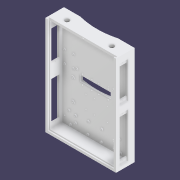
# Autodesk Inventor part: BP001b
Saved by Autodesk Inventor 2017 SP1 (Build 210196100, 196)
## iProperties
Created: 2017-12-18
Part Number: BP001b
Material: ABS Plastic
Document SubType Name: Modeling
Designer: Zach
Density: 1.06 g/cm^3
Appearance: CR White
Author: Zach
Autodesk Inventor part; units mm, degrees
ref_plane "YZ Plane" through (0, 0, 0) normal (1, 0, 0) x (0, 1, 0)
ref_plane "XZ Plane" through (0, 0, 0) normal (0, 1, 0) x (-1, 0, 0)
ref_plane "XY Plane" through (0, 0, 0) normal (0, 0, 1) x (1, 0, 0)
sketch "Sketch1" plane through (0, 0, 0) normal (0, 0, 1) x (1, 0, 0)
  line L0 (0, 0) -> (130, 0)
  line L1 (130, 0) -> (130, 25)
  line L2 (130, 25) -> (0, 25)
  line L3 (0, 25) -> (0, 0)
  line L4 (10.3559, 32.5) -> (50.3559, 32.5) construction
  line L5 (50.3559, 32.5) -> (50.3559, -7.5) construction
  line L6 (50.3559, -7.5) -> (10.3559, -7.5) construction
  line L7 (10.3559, -7.5) -> (10.3559, 32.5) construction
  line L8 (79.6441, 32.5) -> (119.6441, 32.5) construction
  line L9 (119.6441, 32.5) -> (119.6441, -7.5) construction
  line L10 (119.6441, -7.5) -> (79.6441, -7.5) construction
  line L11 (79.6441, -7.5) -> (79.6441, 32.5) construction
  line L12 (50.3559, 12.5) -> (79.6441, 12.5) construction
  circle A0 centre (10.3559, 32.5) radius 2.5
  circle A1 centre (50.3559, 32.5) radius 2.5
  circle A2 centre (50.3559, -7.5) radius 2.5
  circle A3 centre (10.3559, -7.5) radius 2.5
  circle A4 centre (79.6441, -7.5) radius 2.5
  circle A5 centre (119.6441, -7.5) radius 2.5
  circle A6 centre (119.6441, 32.5) radius 2.5
  circle A7 centre (79.6441, 32.5) radius 2.5
  line L13 (-85, -197.5) -> (215, -197.5)
  line L14 (215, -197.5) -> (215, 222.5)
  line L15 (215, 222.5) -> (-85, 222.5)
  line L16 (-85, 222.5) -> (-85, -197.5)
  point P0 (130, 12.5)
  point P1 (65, 12.5)
  point P2 (65, 25)
  point P3 (215, 12.5)
  point P4 (65, 222.5)
  dimension "d0" = 130
  dimension "d1" = 25
  dimension "d2" = 40
  dimension "d3" = 40
  dimension "d4" = 40
  dimension "d5" = 40
  dimension "d6" = 29.2883
  dimension "d7" = 5
  dimension "d8" = 5
  dimension "d9" = 5
  dimension "d10" = 5
  dimension "d11" = 5
  dimension "d12" = 5
  dimension "d13" = 5
  dimension "d14" = 5
  dimension "d15" = 300
  dimension "d16" = 420
  constraints: 34 end point, 8 centre point, 8 coincident, 8 parallel, 7 midpoint, 4 horizontal, 4 perpendicular, 2 horizontal alignment, 2 vertical alignment, 1 point on line
  measures "d0" distance of L2.end L1.end
  measures "d1" distance of L1.end L0.end
  measures "d2" distance of L5.end L6.end
  measures "d3" distance of L4.end L5.end
  measures "d4" distance of L9.end L10.end
  measures "d5" distance of L8.end L9.end
  measures "d6" distance between parallel lines of L11 L5
  measures "d7" diameter of A0
  measures "d8" diameter of A1
  measures "d9" diameter of A2
  measures "d10" diameter of A3
  measures "d11" diameter of A4
  measures "d12" diameter of A5
  measures "d13" diameter of A6
  measures "d14" diameter of A7
  measures "d15" distance of L15.end L14.end
  measures "d16" distance of L14.end L13.end
extrude "Extrusion1" add sketch "Sketch1" along normal blind 17
sketch "Sketch2" plane through (0, 0, 17) normal (0, 0, 1) x (1, 0, 0)
  line L0 (-85, 222.5) -> (-85, -197.5) projected
  line L1 (215, 222.5) -> (-85, 222.5) projected
  line L2 (215, -197.5) -> (215, 222.5) projected
  line L3 (-85, -197.5) -> (215, -197.5) projected
  line L4 (-75, -187.5) -> (-75, 212.5)
  line L5 (-75, 212.5) -> (205, 212.5)
  line L6 (205, 212.5) -> (205, -187.5)
  line L7 (205, -187.5) -> (-75, -187.5)
  point P0 (0, 0)
  dimension "d19" = 10
  constraints: 8 end point, 3 other
  measures "d19" distance between parallel lines of L0 L4
extrude "Extrusion2" add sketch "Sketch2" along normal blind 52
sketch "Sketch3" plane through (-85, 222.5, 0) normal (0, 1, 0) x (1, 0, 0)
  line L0 (0, 0) -> (300, 0) construction
  line L1 (70, 0) -> (230, 0)
  arc A0 (70, 0) -> (230, 0) centre (150, 304.672) ccw
  point P0 (85, 0)
  point P1 (150, 0)
  dimension "d23" = 160
  dimension "d24" = 315
  constraints: 2 end point, 2 midpoint, 2 point on circle, 2 point on line, 1 centre point
  measures "d23" distance of L1.start L1.end
  measures "d24" radius of A0
extrude "Extrusion3" cut sketch "Sketch3" against normal through all
sketch "Sketch5" plane through (0, 0, 17) normal (0, 0, 1) x (1, 0, 0)
  line L0 (-12.46, 197.48) -> (142.46, 197.48) construction
  line L1 (142.46, 197.48) -> (142.46, 40) construction
  line L2 (142.46, 40) -> (-12.46, 40) construction
  line L3 (-12.46, 40) -> (-12.46, 197.48) construction
  line L4 (0, 25) -> (130, 25) construction
  line L5 (-75, 212.5) -> (205, 212.5) construction
  circle A0 centre (142.46, 197.48) radius 1.5
  circle A1 centre (142.46, 40) radius 1.5
  circle A2 centre (-12.46, 40) radius 1.5
  circle A3 centre (-12.46, 197.48) radius 1.5
  circle A4 centre (25.3559, -90.75) radius 1.5
  circle A5 centre (25.3559, -34.25) radius 1.5
  line L6 (130, 0) -> (0, 0) construction
  line L7 (65, 0) -> (65, -187.5) construction
  line L8 (-75, -187.5) -> (205, -187.5) projected
  line L9 (-75, -187.5) -> (-75, 212.5) projected
  line L10 (205, 212.5) -> (205, -187.5) projected
  line L11 (160, -90) -> (160, 0) construction
  circle A6 centre (160, 0) radius 1.5
  circle A7 centre (160, -90) radius 1.5
  line L12 (-30, 0) -> (-30, -90) construction
  circle A8 centre (-30, 0) radius 1.5
  circle A9 centre (-30, -90) radius 1.5
  circle A10 centre (119.62, 40) radius 1.5
  line L13 (60.3559, -92.5) -> (116.8559, -92.5) construction
  circle A11 centre (116.8559, -92.5) radius 1.5
  circle A12 centre (60.3559, -92.5) radius 1.5
  line L14 (60.3559, -32.5) -> (116.8559, -32.5) construction
  circle A13 centre (116.8559, -32.5) radius 1.5
  circle A14 centre (60.3559, -32.5) radius 1.5
  circle A15 centre (50.3559, -7.5) radius 2.5 construction
  line L15 (25.3559, -34.25) -> (25.3559, -90.75) construction
  line L16 (88.6059, -92.5) -> (88.6059, -32.5) construction
  point P0 (65, 40)
  point P1 (65, -93.75)
  point P2 (65, -80)
  point P3 (88.6059, -62.5)
  point P4 (25.3559, -62.5)
  dimension "d27" = 154.92
  dimension "d28" = 157.48
  dimension "d29" = 3
  dimension "d30" = 3
  dimension "d31" = 3
  dimension "d32" = 3
  dimension "d34" = 3
  dimension "d35" = 3
  dimension "d112" = 45
  dimension "d115" = 3
  dimension "d116" = 3
  dimension "d117" = 45
  dimension "d118" = 3
  dimension "d119" = 3
  dimension "d129" = 90
  dimension "d131" = 0
  dimension "d239" = 3
  dimension "d240" = 22.84
  dimension "d241" = 15
  dimension "d260" = 56.5
  dimension "d261" = 3
  dimension "d262" = 3
  dimension "d263" = 56.5
  dimension "d264" = 3
  dimension "d265" = 3
  dimension "d266" = 10
  dimension "d267" = 25
  dimension "d268" = 60
  dimension "d269" = 56.5
  dimension "d270" = 35
  constraints: 22 end point, 15 centre point, 12 coincident, 11 midpoint, 4 vertical alignment, 3 horizontal, 3 horizontal alignment, 3 vertical, 2 parallel, 1 perpendicular, 1 point on line
  measures "d27" distance of L1.end L2.end
  measures "d28" distance of L0.end L1.end
  measures "d29" diameter of A0
  measures "d30" diameter of A1
  measures "d31" diameter of A2
  measures "d32" diameter of A3
  measures "d34" diameter of A4
  measures "d35" diameter of A5
  measures "d112" distance between parallel lines of L10 L11
  measures "d115" diameter of A6
  measures "d116" diameter of A7
  measures "d117" distance between parallel lines of L9 L12
  measures "d118" diameter of A8
  measures "d119" diameter of A9
  measures "d129" distance of A6.centre L11.start
  measures "d131" distance from line of L11.end L6
  measures "d239" diameter of A10
  measures "d240" distance from line of L1 A10.centre
  measures "d241" distance between parallel lines of L4 L2
  measures "d260" distance of L13.start L13.end
  measures "d261" diameter of A11
  measures "d262" diameter of A12
  measures "d263" distance of L14.start L14.end
  measures "d264" diameter of A13
  measures "d265" diameter of A14
  measures "d266" horizontal distance of A15.centre L14.start
  measures "d267" vertical distance of A15.centre L14.end
  measures "d268" distance between parallel lines of L13 L14
  measures "d269" distance of L15.end L15.start
  measures "d270" distance from line of L14.start L15
extrude "Extrusion4" cut sketch "Sketch5" against normal through all
sketch "Sketch6" plane through (0, 0, 17) normal (0, 0, 1) x (1, 0, 0)
  circle A0 centre (-12.46, 197.48) radius 1.5 projected
  line L0 (205, 212.5) -> (-75, 212.5) projected
  line L1 (-75, 212.5) -> (-75, -187.5) projected
  line L2 (-75, -187.5) -> (205, -187.5) projected
  line L3 (205, -187.5) -> (205, 212.5) projected
  line L4 (0, 0) -> (0, 25) projected
  line L5 (0, 25) -> (130, 25) projected
  line L6 (130, 25) -> (130, 0) projected
  line L7 (130, 0) -> (0, 0) projected
  circle A1 centre (79.6441, 32.5) radius 2.5 projected
  circle A2 centre (119.6441, 32.5) radius 2.5 projected
  circle A3 centre (119.6441, -7.5) radius 2.5 projected
  circle A4 centre (79.6441, -7.5) radius 2.5 projected
  circle A5 centre (10.3559, -7.5) radius 2.5 projected
  circle A6 centre (50.3559, -7.5) radius 2.5 projected
  circle A7 centre (50.3559, 32.5) radius 2.5 projected
  circle A8 centre (10.3559, 32.5) radius 2.5 projected
  circle A9 centre (-12.46, 197.48) radius 5
  circle A10 centre (142.46, 197.48) radius 1.5 projected
  circle A11 centre (142.46, 197.48) radius 5
  circle A12 centre (142.46, 40) radius 5
  circle A13 centre (-12.46, 40) radius 1.5 projected
  circle A14 centre (-12.46, 40) radius 5
  circle A15 centre (142.46, 40) radius 1.5 projected
  circle A16 centre (-30, 0) radius 1.5 projected
  circle A17 centre (-30, -90) radius 1.5 projected
  circle A18 centre (160, 0) radius 1.5 projected
  circle A19 centre (160, -90) radius 1.5 projected
  circle A20 centre (-30, 0) radius 1.5 projected
  circle A21 centre (-30, 0) radius 7.5
  circle A22 centre (-30, -90) radius 7.5
  circle A23 centre (160, 0) radius 7.5
  circle A24 centre (160, -90) radius 7.5
  circle A25 centre (119.62, 40) radius 1.5 projected
  circle A26 centre (119.62, 40) radius 5
  dimension "d58" = 10
  dimension "d59" = 10
  dimension "d60" = 10
  dimension "d61" = 10
  dimension "d120" = 15
  dimension "d121" = 15
  dimension "d122" = 15
  dimension "d123" = 15
  dimension "d242" = 10
  constraints: 9 centre point, 9 coincident
  measures "d58" diameter of A9
  measures "d59" diameter of A11
  measures "d60" diameter of A12
  measures "d61" diameter of A14
  measures "d120" diameter of A21
  measures "d121" diameter of A22
  measures "d122" diameter of A23
  measures "d123" diameter of A24
  measures "d242" diameter of A26
extrude "Extrusion5" add sketch "Sketch6" along normal blind 3 contours A9 | A11 | A12 | A14 | A21 | A22 | A23 | A24
sketch "Sketch7" plane through (-75, -187.5, 17) normal (1, 0, 0) x (0, 0, -1)
  line L0 (-3, 389.98) -> (-3, 379.98) projected
  line L1 (-3, 232.5) -> (-3, 222.5) projected
  line L2 (-3, 379.98) -> (-3, 232.5)
  line L3 (-12, 368.24) -> (-47, 368.24)
  line L4 (-47, 368.24) -> (-47, 244.24)
  line L5 (-47, 244.24) -> (-12, 244.24)
  line L6 (-12, 244.24) -> (-12, 368.24)
  line L7 (0, 180) -> (0, 195) projected
  line L8 (0, 180) -> (0, 195) projected
  line L9 (0, 222.5) -> (0, 232.5) projected
  line L10 (0, 379.98) -> (0, 389.98) projected
  line L11 (0, 379.98) -> (0, 389.98) projected
  line L12 (0, 222.5) -> (0, 232.5) projected
  line L13 (0, 90) -> (0, 105) projected
  line L14 (0, 90) -> (0, 105) projected
  line L15 (0, 400) -> (0, 0) projected
  line L16 (0, 0) -> (0, 400) projected
  line L17 (0, 187.5) -> (0, 212.5) projected
  line L18 (0, 212.5) -> (0, 187.5) projected
  line L19 (0, 217.5) -> (0, 222.5) projected
  line L20 (0, 217.5) -> (0, 222.5) projected
  line L21 (0, 177.5) -> (0, 182.5) projected
  line L22 (0, 177.5) -> (0, 182.5) projected
  line L23 (0, 177.5) -> (0, 182.5) projected
  line L24 (0, 177.5) -> (0, 182.5) projected
  line L25 (0, 217.5) -> (0, 222.5) projected
  line L26 (0, 217.5) -> (0, 222.5) projected
  line L27 (17, 410) -> (17, -10) projected
  point P0 (17, 187.5)
  point P1 (-47, 306.24)
  point P2 (-3, 306.24)
  point P3 (0, 106)
  point P4 (0, 109)
  point P5 (0, 106)
  point P6 (0, 109)
  point P7 (0, 146)
  point P8 (0, 149)
  point P9 (0, 146)
  point P10 (0, 149)
  point P11 (0, 98)
  point P12 (0, 101)
  point P13 (0, 98)
  point P14 (0, 101)
  dimension "d124" = 35
  dimension "d125" = 124
  dimension "d259" = 29
  constraints: 10 end point, 2 midpoint, 2 parallel, 1 horizontal, 1 horizontal alignment, 1 perpendicular, 1 vertical
  measures "d124" distance of L5.end L4.end
  measures "d125" distance of L4.end L3.end
  measures "d259" distance between parallel lines of L27 L6
extrude "Extrusion6" cut sketch "Sketch7" against normal through all
sketch "Sketch8" plane through (-85, -197.5, 0) normal (-1, 0, 0) x (0, 0, 1)
  line L0 (64, 378.24) -> (29, 378.24)
  line L1 (29, 378.24) -> (29, 393.24)
  line L2 (29, 393.24) -> (64, 393.24)
  line L3 (64, 393.24) -> (64, 378.24)
  line L4 (64, 254.24) -> (29, 254.24)
  line L5 (29, 254.24) -> (29, 239.24)
  line L6 (29, 239.24) -> (64, 239.24)
  line L7 (64, 239.24) -> (64, 254.24)
  line L8 (29, 378.24) -> (64, 378.24) projected
  line L9 (64, 254.24) -> (29, 254.24) projected
  line L10 (29, 254.24) -> (29, 378.24) projected
  point P0 (0, 187.5)
  point P1 (29, 385.74)
  point P2 (29, 246.74)
  dimension "d73" = 15
  dimension "d74" = 15
  constraints: 16 end point, 4 parallel, 2 horizontal, 2 midpoint, 2 perpendicular, 1 vertical alignment
  measures "d73" distance of L0.end L1.end
  measures "d74" distance of L4.end L5.end
extrude "Extrusion7" cut sketch "Sketch8" against normal blind 5
sketch "Sketch9" plane through (-80, -197.5, 0) normal (-1, 0, 0) x (0, 0, 1)
  circle A0 centre (46.5, 246.74) radius 1.5
  line L0 (29, 239.24) -> (29, 254.24) projected
  line L1 (64, 239.24) -> (29, 239.24) projected
  line L2 (64, 254.24) -> (64, 239.24) projected
  line L3 (29, 393.24) -> (64, 393.24) projected
  line L4 (64, 393.24) -> (64, 378.24) projected
  line L5 (29, 393.24) -> (64, 393.24) projected
  line L6 (29, 378.24) -> (29, 393.24) projected
  circle A1 centre (46.5, 385.74) radius 1.5
  line L7 (64, 378.24) -> (29, 378.24) projected
  line L8 (29, 254.24) -> (64, 254.24) projected
  line L9 (64, 378.24) -> (29, 378.24) projected
  point P0 (0, 197.5)
  point P1 (29, 246.74)
  point P2 (29, 385.74)
  point P3 (46.5, 378.24)
  point P4 (46.5, 254.24)
  point P5 (46.5, 378.24)
  dimension "d77" = 3
  dimension "d78" = 3
  constraints: 4 midpoint, 3 vertical alignment, 2 centre point, 2 horizontal alignment
  measures "d77" diameter of A0
  measures "d78" diameter of A1
extrude "Extrusion8" cut sketch "Sketch9" against normal through all contours A0 | A1
sketch "Sketch10" plane through (215, -197.5, 0) normal (1, 0, 0) x (0, 0, -1)
  circle A0 centre (-46.5, 246.74) radius 1.5 projected
  line L0 (-29, 239.24) -> (-29, 254.24) projected
  line L1 (-64, 239.24) -> (-29, 239.24) projected
  line L2 (-64, 254.24) -> (-64, 239.24) projected
  line L3 (-29, 254.24) -> (-64, 254.24) projected
  circle A1 centre (-46.5, 385.74) radius 1.5 projected
  line L4 (-29, 378.24) -> (-29, 393.24) projected
  line L5 (-64, 378.24) -> (-29, 378.24) projected
  line L6 (-64, 393.24) -> (-64, 378.24) projected
  line L7 (-29, 393.24) -> (-64, 393.24) projected
  point P0 (0, 187.5)
extrude "Extrusion9" cut sketch "Sketch10" against normal blind 5
sketch "Sketch13" plane through (205, -187.5, 17) normal (-1, 0, 0) x (0, 0, 1)
  line L0 (47, 368.24) -> (12, 368.24) projected
  line L1 (47, 383.24) -> (47, 229.24) projected
  line L2 (12, 229.24) -> (12, 383.24) projected
  line L3 (12, 244.24) -> (47, 244.24) projected
  line L4 (12, 368.24) -> (47, 368.24)
  line L5 (47, 368.24) -> (47, 244.24)
  line L6 (47, 244.24) -> (12, 244.24)
  line L7 (12, 244.24) -> (12, 368.24)
  constraints: 8 end point, 2 parallel, 1 horizontal, 1 perpendicular
extrude "Extrusion12" cut sketch "Sketch13" against normal through all
sketch "Sketch14" plane through (-85, 222.5, 69) normal (0, 1, 0) x (1, 0, 0)
  line L0 (290, 52) -> (10, 52) projected
  circle A0 centre (55, 27) radius 10
  line L1 (150, 52) -> (150, -9.8542)
  circle A1 centre (245, 27) radius 10
  point P0 (85, 69)
  dimension "d99" = 20
  dimension "d100" = 25
  dimension "d103" = 95
  dimension "d279" = 20
  dimension "d280" = 95
  constraints: 2 centre point, 2 end point, 1 horizontal alignment, 1 midpoint, 1 vertical
  measures "d99" diameter of A0
  measures "d100" distance from line of L0 A0.centre
  measures "d103" distance from line of L1 A0.centre
  measures "d279" diameter of A1
  measures "d280" distance from line of A1.centre L1
extrude "Extrusion13" cut sketch "Sketch14" against normal blind 25
sketch "Sketch18" plane through (0, 0, 17) normal (0, 0, 1) x (1, 0, 0)
  circle A0 centre (174, -176.5) radius 1.5
  circle A1 centre (146, -171) radius 1.5
  circle A2 centre (146, -143.6) radius 1.5
  circle A3 centre (167.5, -128.1) radius 1.5
  circle A4 centre (93.5, -128.1) radius 1.5
  circle A5 centre (92, -176.5) radius 1.5
  line L0 (205, -187.5) -> (-75, -187.5) projected
  line L1 (205, 212.5) -> (205, -187.5) projected
  circle A6 centre (-17.5, -133.6) radius 1.5
  circle A7 centre (-17.5, -161) radius 1.5
  circle A8 centre (35, -176.5) radius 1.5
  circle A9 centre (36.5, -128.1) radius 1.5
  circle A10 centre (-39, -176.5) radius 1.5
  circle A11 centre (-45.5, -128.1) radius 1.5
  line L2 (-75, -187.5) -> (-75, 212.5) projected
  line L3 (130, 0) -> (0, 0) projected
  line L4 (65, 0) -> (65, -187.5) construction
  line L5 (36.5, -128.1) -> (65, -128.1) construction
  line L6 (93.5, -128.1) -> (65, -128.1) construction
  dimension "d169" = 82
  dimension "d170" = 48.4
  dimension "d171" = 1.5
  dimension "d172" = 15.5
  dimension "d173" = 27.4
  dimension "d174" = 48.4
  dimension "d175" = 6.5
  dimension "d176" = 74
  dimension "d177" = 5.5
  dimension "d178" = 28
  dimension "d179" = 3
  dimension "d180" = 3
  dimension "d181" = 3
  dimension "d182" = 3
  dimension "d183" = 3
  dimension "d184" = 3
  dimension "d185" = 11
  dimension "d186" = 31
  dimension "d189" = 82
  dimension "d190" = 48.4
  dimension "d191" = 1.5
  dimension "d192" = 15.5
  dimension "d193" = 27.4
  dimension "d194" = 48.4
  dimension "d195" = 6.5
  dimension "d196" = 74
  dimension "d197" = 5.5
  dimension "d198" = 28
  dimension "d199" = 3
  dimension "d200" = 3
  dimension "d201" = 3
  dimension "d202" = 3
  dimension "d203" = 3
  dimension "d204" = 3
  constraints: 12 centre point, 6 end point, 2 coincident, 2 midpoint, 1 collinear, 1 horizontal alignment, 1 perpendicular, 1 point on line
  measures "d169" distance of A5.centre A0.centre
  measures "d170" vertical distance of L6.start A5.centre
  measures "d171" horizontal distance of A5.centre L6.start
  measures "d172" vertical distance of A2.centre L6.start
  measures "d173" distance of A1.centre A2.centre
  measures "d174" vertical distance of A3.centre A0.centre
  measures "d175" horizontal distance of A0.centre A3.centre
  measures "d176" distance of L6.start A3.centre
  measures "d177" vertical distance of A1.centre A0.centre
  measures "d178" horizontal distance of A0.centre A1.centre
  measures "d179" diameter of A0
  measures "d180" diameter of A3
  measures "d181" diameter of A2
  measures "d182" diameter of A1
  measures "d183" diameter of A5
  measures "d184" diameter of A4
  measures "d185" distance from line of L0 A0.centre
  measures "d186" distance from line of A0.centre L1
  measures "d189" distance of A9.centre A11.centre
  measures "d190" vertical distance of A8.centre A9.centre
  measures "d191" horizontal distance of A9.centre A8.centre
  measures "d192" vertical distance of A7.centre A8.centre
  measures "d193" distance of A6.centre A7.centre
  measures "d194" vertical distance of A10.centre A11.centre
  measures "d195" horizontal distance of A11.centre A10.centre
  measures "d196" distance of A8.centre A10.centre
  measures "d197" vertical distance of A6.centre A11.centre
  measures "d198" horizontal distance of A11.centre A6.centre
  measures "d199" diameter of A11
  measures "d200" diameter of A10
  measures "d201" diameter of A7
  measures "d202" diameter of A6
  measures "d203" diameter of A9
  measures "d204" diameter of A8
extrude "Extrusion16" cut sketch "Sketch18" against normal through all
sketch "Sketch20" plane through (0, 0, 69) normal (0, 0, 1) x (1, 0, 0)
  line L0 (-85, 222.5) -> (-85, -197.5) projected
  line L1 (-85, -197.5) -> (215, -197.5) projected
  line L2 (215, -197.5) -> (215, 222.5) projected
  line L3 (-80, 222.5) -> (-80, -192.5)
  line L4 (-80, -192.5) -> (210, -192.5)
  line L5 (210, -192.5) -> (210, 222.5)
  line L6 (215, 222.5) -> (-85, 222.5) projected
  line L7 (-85, 222.5) -> (-80, 222.5)
  line L8 (215, 222.5) -> (210, 222.5)
  point P0 (0, 0)
  dimension "d214" = 5
  constraints: 10 end point, 2 collinear, 2 other
  measures "d214" distance between parallel lines of L0 L3
extrude "Extrusion18" add sketch "Sketch20" along normal blind 5 contours L6 L3 L4 L5 L2 L1 L0
sketch "Sketch21" plane through (0, 0, 74) normal (0, 0, 1) x (1, 0, 0)
  line L0 (-80, -192.5) -> (-80, 222.5) projected
  line L1 (215, -197.5) -> (215, 222.5) projected
  line L2 (210, 222.5) -> (210, -192.5) projected
  line L3 (-85, 222.5) -> (-85, -197.5) projected
  line L4 (-85, 222.5) -> (-85, -197.5) projected
  line L5 (-85, -197.5) -> (215, -197.5) projected
  line L6 (215, -197.5) -> (215, 222.5) projected
  line L7 (215, 222.5) -> (210, 222.5) projected
  line L8 (210, 222.5) -> (210, -192.5) projected
  line L9 (210, -192.5) -> (-80, -192.5) projected
  line L10 (-80, -192.5) -> (-80, 222.5) projected
  line L11 (-80, 222.5) -> (-85, 222.5) projected
  line L12 (-75, -187.5) -> (-75, 212.5) projected
  line L13 (205, 212.5) -> (205, -187.5) projected
  line L14 (205, -187.5) -> (-75, -187.5) projected
  line L15 (-75, -187.5) -> (-75, -192.5)
  line L16 (205, -187.5) -> (205, -192.5)
  line L17 (-75, 212.5) -> (-75, 222.5)
  line L18 (210, 222.5) -> (-80, 222.5) projected
  line L19 (-75, 222.5) -> (-80, 222.5)
  line L20 (205, 212.5) -> (205, 222.5)
  line L21 (215, 222.5) -> (210, 222.5) projected
  line L22 (205, 222.5) -> (210, 222.5)
  line L23 (-80, -192.5) -> (210, -192.5) projected
  line L24 (205, -192.5) -> (210, -192.5)
  line L25 (-75, -192.5) -> (-80, -192.5)
  point P0 (0, 0)
  constraints: 16 end point, 5 point on line, 3 collinear, 3 perpendicular, 1 horizontal
extrude "Extrusion19" add sketch "Sketch21" along normal blind 5 contours L9 L2 L7 L1 L5 L3 L11 L0 | L0 L18 L17 L12 L15 L9 | L15 L14 L16 L9 | L16 L13 L20 L18 L2 L9
sketch "Sketch22" plane through (0, 0, 69) normal (0, 0, 1) x (1, 0, 0)
  circle A0 centre (65, 217.5) radius 2.5
  line L0 (210, 222.5) -> (-80, 222.5) projected
  point P0 (0, 0)
  point P1 (65, 222.5)
  dimension "d219" = 5
  dimension "d220" = 5
  constraints: 1 centre point, 1 midpoint, 1 vertical alignment
  measures "d219" diameter of A0
  measures "d220" distance from line of L0 A0.centre
extrude "Extrusion20" cut sketch "Sketch22" against normal blind 25
sketch "Sketch23" plane through (215, -197.5, 0) normal (1, 0, 0) x (0, 0, -1)
  line L0 (-64, 239.24) -> (-64, 393.24) projected
  line L1 (-29, 393.24) -> (-29, 239.24) projected
  line L2 (-64, 192.5) -> (-29, 192.5)
  line L3 (-29, 192.5) -> (-29, 32.5)
  line L4 (-29, 32.5) -> (-64, 32.5)
  line L5 (-64, 32.5) -> (-64, 192.5)
  point P0 (0, 197.5)
  dimension "d223" = 160
  dimension "d224" = 5
  constraints: 8 end point, 2 parallel, 2 vertical alignment, 1 horizontal, 1 perpendicular
  measures "d223" distance of L2.end L3.end
  measures "d224" vertical distance of point (0, 197.5) L2.end
extrude "Extrusion21" cut sketch "Sketch23" against normal blind 10
sketch "Sketch24" plane through (-85, -197.5, 0) normal (-1, 0, 0) x (0, 0, 1)
  line L0 (64, 192.5) -> (29, 192.5) projected
  line L1 (29, 192.5) -> (29, 32.5) projected
  line L2 (64, 32.5) -> (64, 192.5) projected
  line L3 (29, 32.5) -> (64, 32.5) projected
  point P0 (0, 197.5)
extrude "Extrusion22" cut sketch "Sketch24" against normal blind 10
sketch "Sketch25" plane through (210, -197.5, 0) normal (1, 0, 0) x (0, 0, -1)
  line L0 (-29, 192.5) -> (-64, 192.5) projected
  line L1 (-64, 192.5) -> (-29, 192.5)
  line L2 (-29, 192.5) -> (-29, 207.5)
  line L3 (-29, 207.5) -> (-64, 207.5)
  line L4 (-64, 207.5) -> (-64, 192.5)
  line L5 (-29, 32.5) -> (-29, 192.5) projected
  line L6 (-64, 32.5) -> (-29, 32.5) projected
  line L7 (-64, 32.5) -> (-29, 32.5)
  line L8 (-29, 32.5) -> (-29, 17.5)
  line L9 (-29, 17.5) -> (-64, 17.5)
  line L10 (-64, 17.5) -> (-64, 32.5)
  point P0 (0, 197.5)
  dimension "d229" = 15
  dimension "d230" = 15
  constraints: 16 end point, 4 parallel, 2 horizontal, 2 perpendicular
  measures "d229" distance of L0.start L2.end
  measures "d230" distance of L5.start L8.end
extrude "Extrusion23" cut sketch "Sketch25" along normal through all
sketch "Sketch26" plane through (-80, -197.5, 0) normal (-1, 0, 0) x (0, 0, 1)
  line L0 (29, 192.5) -> (29, 207.5) projected
  line L1 (29, 207.5) -> (64, 207.5) projected
  line L2 (64, 207.5) -> (64, 192.5) projected
  line L3 (29, 192.5) -> (64, 192.5) projected
  line L4 (64, 32.5) -> (29, 32.5) projected
  line L5 (64, 32.5) -> (64, 17.5) projected
  line L6 (64, 17.5) -> (29, 17.5) projected
  line L7 (29, 17.5) -> (29, 32.5) projected
  point P0 (0, 197.5)
extrude "Extrusion24" cut sketch "Sketch26" along normal through all
sketch "Sketch27" plane through (-80, -197.5, 0) normal (-1, 0, 0) x (0, 0, 1)
  line L0 (29, 32.5) -> (64, 32.5) construction
  line L1 (29, 17.5) -> (29, 32.5) construction
  line L2 (64, 17.5) -> (29, 17.5) construction
  line L3 (64, 32.5) -> (64, 17.5) construction
  line L4 (29, 192.5) -> (29, 207.5) construction
  line L5 (64, 192.5) -> (29, 192.5) construction
  line L6 (64, 207.5) -> (64, 192.5) construction
  line L7 (29, 207.5) -> (64, 207.5) construction
  circle A0 centre (46.5, 200) radius 1.5
  circle A1 centre (46.5, 25) radius 1.5
  point P0 (0, 197.5)
  point P1 (29, 200)
  point P2 (46.5, 207.5)
  point P3 (46.5, 32.5)
  point P4 (29, 25)
  dimension "d235" = 3
  dimension "d236" = 3
  constraints: 4 midpoint, 2 centre point, 2 horizontal alignment, 2 vertical alignment
  measures "d235" diameter of A0
  measures "d236" diameter of A1
extrude "Extrusion25" cut sketch "Sketch27" against normal through all
sketch "Sketch29" plane through (0, 0, 17) normal (0, 0, 1) x (1, 0, 0)
  circle A0 centre (-45.5, -128.1) radius 1.5 projected
  circle A1 centre (-17.5, -133.6) radius 1.5 projected
  circle A2 centre (-17.5, -161) radius 1.5 projected
  circle A3 centre (-39, -176.5) radius 1.5 projected
  circle A4 centre (35, -176.5) radius 1.5 projected
  circle A5 centre (36.5, -128.1) radius 1.5 projected
  circle A6 centre (93.5, -128.1) radius 1.5 projected
  circle A7 centre (92, -176.5) radius 1.5 projected
  circle A8 centre (146, -171) radius 1.5 projected
  circle A9 centre (146, -143.6) radius 1.5 projected
  circle A10 centre (167.5, -128.1) radius 1.5 projected
  circle A11 centre (174, -176.5) radius 1.5 projected
  circle A12 centre (-17.5, -133.6) radius 5
  circle A13 centre (-45.5, -128.1) radius 5
  circle A14 centre (-39, -176.5) radius 5
  circle A15 centre (-17.5, -161) radius 5
  circle A16 centre (35, -176.5) radius 5
  circle A17 centre (36.5, -128.1) radius 5
  circle A18 centre (93.5, -128.1) radius 5
  circle A19 centre (92, -176.5) radius 5
  circle A20 centre (146, -143.6) radius 5
  circle A21 centre (146, -171) radius 5
  circle A22 centre (174, -176.5) radius 5
  circle A23 centre (167.5, -128.1) radius 5
  point P0 (0, 0)
  dimension "d245" = 10
  dimension "d246" = 10
  dimension "d247" = 10
  dimension "d248" = 10
  dimension "d249" = 10
  dimension "d250" = 10
  dimension "d251" = 10
  dimension "d252" = 10
  dimension "d253" = 10
  dimension "d254" = 10
  dimension "d255" = 10
  dimension "d256" = 10
  constraints: 12 centre point, 12 coincident
  measures "d245" diameter of A12
  measures "d246" diameter of A13
  measures "d247" diameter of A14
  measures "d248" diameter of A15
  measures "d249" diameter of A16
  measures "d250" diameter of A17
  measures "d251" diameter of A18
  measures "d252" diameter of A19
  measures "d253" diameter of A20
  measures "d254" diameter of A21
  measures "d255" diameter of A22
  measures "d256" diameter of A23
extrude "Extrusion27" add sketch "Sketch29" along normal blind 5
sketch "Sketch30" plane through (0, 0, 17) normal (0, 0, 1) x (1, 0, 0)
  circle A0 centre (-65, -157) radius 2.5
  line L0 (-75, -187.5) -> (-75, 222.5) projected
  line L1 (205, -187.5) -> (-75, -187.5) projected
  circle A1 centre (195, -157) radius 2.5
  line L2 (205, 222.5) -> (205, -187.5) projected
  point P0 (0, 0)
  dimension "d271" = 5
  dimension "d272" = 10
  dimension "d273" = 30.5
  dimension "d274" = 5
  dimension "d275" = 10
  dimension "d276" = 30.5
  constraints: 2 centre point
  measures "d271" diameter of A0
  measures "d272" distance from line of L0 A0.centre
  measures "d273" distance from line of L1 A0.centre
  measures "d274" diameter of A1
  measures "d275" distance from line of L2 A1.centre
  measures "d276" distance from line of L1 A1.centre
extrude "Extrusion28" cut sketch "Sketch30" against normal through all
sketch "Sketch31" plane through (0, 0, 17) normal (0, 0, 1) x (1, 0, 0)
  line L0 (-65, 86.5) -> (-28, 86.5) construction
  line L1 (-28, 86.5) -> (-28, 33.5) construction
  line L2 (-28, 33.5) -> (-65, 33.5) construction
  line L3 (-65, 33.5) -> (-65, 86.5) construction
  circle A0 centre (-28, 86.5) radius 1.5
  circle A1 centre (-65, 86.5) radius 1.5
  circle A2 centre (-28, 33.5) radius 1.5
  circle A3 centre (-65, 33.5) radius 1.5
  line L4 (-75, 212.5) -> (-75, -187.5) projected
  line L5 (-75, 56.74) -> (-80, 56.74) projected
  line L6 (205, 212.5) -> (-75, 212.5) projected
  point P0 (0, 0)
  dimension "d281" = 3
  dimension "d282" = 3
  dimension "d283" = 3
  dimension "d284" = 3
  dimension "d286" = 10
  dimension "d287" = 53
  dimension "d288" = 37
  dimension "d292" = 126
  constraints: 8 end point, 4 centre point, 4 coincident, 2 parallel, 1 horizontal, 1 perpendicular
  measures "d281" diameter of A0
  measures "d282" diameter of A1
  measures "d283" diameter of A2
  measures "d284" diameter of A3
  measures "d286" distance from line of L4 L2.end
  measures "d287" distance of L2.end L0.start
  measures "d288" distance of L0.start L0.end
  measures "d292" distance from line of L6 L0.start
extrude "Extrusion29" cut sketch "Sketch31" against normal through all
sketch "Sketch32" plane through (0, 0, 17) normal (0, 0, 1) x (1, 0, 0)
  circle A0 centre (-65, 86.5) radius 1.5 projected
  circle A1 centre (-28, 86.5) radius 1.5 projected
  circle A2 centre (-28, 33.5) radius 1.5 projected
  circle A3 centre (-65, 33.5) radius 1.5 projected
  circle A4 centre (-28, 86.5) radius 5
  circle A5 centre (-65, 86.5) radius 1.5 projected
  circle A6 centre (-65, 86.5) radius 5
  circle A7 centre (-28, 33.5) radius 5
  circle A8 centre (-65, 33.5) radius 5
  point P0 (0, 0)
  dimension "d291" = 10
  dimension "d293" = 10
  dimension "d294" = 10
  dimension "d295" = 10
  constraints: 4 centre point, 4 coincident
  measures "d291" diameter of A4
  measures "d293" diameter of A6
  measures "d294" diameter of A7
  measures "d295" diameter of A8
extrude "Extrusion30" add sketch "Sketch32" along normal blind 3
body "Solid1"
